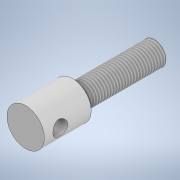
# Autodesk Inventor part: CompressionGripAttachment
Saved by Autodesk Inventor 2020 (Build 240168000, 168)
## iProperties
Created: 2020-03-16
Part Number: CompressionGripAttachment
Material: Generic
Document SubType Name: Modeling
Designer: 19673418
Density: 1 g/cm^3
Appearance: Default
Author: 19673418
Autodesk Inventor part; units mm, degrees
ref_plane "YZ Plane" through (0, 0, 0) normal (1, 0, 0) x (0, 1, 0)
ref_plane "XZ Plane" through (0, 0, 0) normal (0, 1, 0) x (-1, 0, 0)
ref_plane "XY Plane" through (0, 0, 0) normal (0, 0, 1) x (1, 0, 0)
sketch "Sketch1" plane through (0, 0, 0) normal (0, 0, 1) x (1, 0, 0)
  circle A0 centre (0, 0) radius 10
  dimension "d0" = 20
  constraints: 1 centre point, 1 coincident
  measures "d0" diameter of A0
extrude "Extrusion1" add sketch "Sketch1" along normal blind 70
sketch "Sketch2" plane through (0, 0, 70) normal (0, 0, 1) x (1, 0, 0)
  circle A0 centre (0, 0) radius 16
  dimension "d3" = 32
  constraints: 1 centre point, 1 coincident
  measures "d3" diameter of A0
extrude "Extrusion2" add sketch "Sketch2" along normal blind 40
sketch "Sketch3" plane through (0, 0, 0) normal (1, 0, 0) x (0, 1, 0)
  line L0 (16, 70) -> (-16, 70) projected
  point P0 (0, 0)
  point P1 (0, 96.35)
  dimension "d6" = 26.35
  measures "d6" distance from line of L0 point (0, 96.35)
hole "Hole1" at (0, 0, 96.35) direction (-1, 0, 0) diameter 12.7 end through all both
thread "Thread1" size "M20x2.5" class "6g" standard "ANSI Metric M Profile" full length
body "Solid1"
